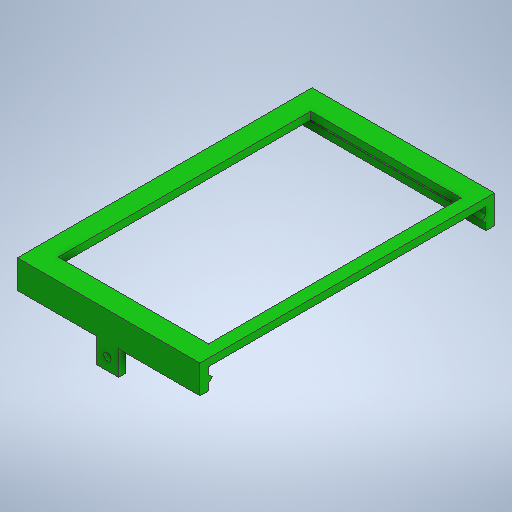
# Autodesk Inventor part: plate top
Saved by Autodesk Inventor 2026.1 (Build 301233020, 233B)
## iProperties
Created: 2025-07-03
Part Number: plate top
Material: Generic
Document SubType Name: Modeling
Designer: admin
Density: 1 g/cm^3
Appearance: Default
Author: admin
Autodesk Inventor part; units mm, degrees
ref_plane "YZ Plane" through (0, 0, 0) normal (1, 0, 0) x (0, 1, 0)
ref_plane "XZ Plane" through (0, 0, 0) normal (0, 1, 0) x (-1, 0, 0)
ref_plane "XY Plane" through (0, 0, 0) normal (0, 0, 1) x (1, 0, 0)
sketch "Sketch1" plane through (0, 0, 0) normal (0, 1, 0) x (-1, 0, 0)
  line L0 (21.9355, 25.495) -> (-52.0645, 25.495)
  line L1 (-52.0645, 25.495) -> (-52.0645, -94.005)
  line L2 (-52.0645, -94.005) -> (21.9355, -94.005)
  line L3 (21.9355, -94.005) -> (21.9355, 25.495)
  point P0 (0, 0)
  dimension "d0" = 119.5
  dimension "d1" = 74
  constraints: 8 end point, 3 perpendicular, 1 horizontal
  measures "d0" distance of L2.end L0.start
  measures "d1" distance of L0.start L0.end
extrude "Extrusion1" add sketch "Sketch1" against normal blind 3
sketch "Sketch2" plane through (0, 0, 0) normal (0, 1, 0) x (1, 0, 0)
  line L0 (-13.9355, -16.995) -> (-13.9355, 85.505)
  line L1 (-13.9355, 85.505) -> (47.0645, 85.505)
  line L2 (-21.9355, 94.005) -> (52.0645, 94.005) projected
  line L3 (47.0645, 85.505) -> (47.0645, -16.995)
  line L4 (47.0645, -16.995) -> (-13.9355, -16.995)
  line L5 (-21.9355, -25.495) -> (52.0645, -25.495) projected
  line L6 (-21.9355, 94.005) -> (-21.9355, -25.495) projected
  line L7 (52.0645, -25.495) -> (52.0645, 94.005) projected
  point P0 (0, 0)
  dimension "d4" = 8.5
  dimension "d5" = 8.5
  dimension "d6" = 8
  dimension "d7" = 5
  constraints: 8 end point, 2 perpendicular, 1 parallel, 1 vertical
  measures "d4" distance between parallel lines of L4 L5
  measures "d5" distance between parallel lines of L1 L2
  measures "d6" distance between parallel lines of L0 L6
  measures "d7" distance between parallel lines of L7 L3
extrude "Extrusion2" cut sketch "Sketch2" against normal blind 3 contours L0 L1 L3 L4
sketch "Sketch7" plane through (0, -3, 0) normal (0, -1, 0) x (1, 0, 0)
  line L0 (52.0645, 25.495) -> (-21.9355, 25.495) projected
  line L1 (52.0645, 25.495) -> (52.0645, 21.995)
  line L2 (52.0645, -94.005) -> (52.0645, 25.495) projected
  line L3 (52.0645, 21.995) -> (-21.9355, 21.995)
  line L4 (-21.9355, 21.995) -> (-21.9355, 25.495)
  line L5 (-21.9355, 25.495) -> (52.0645, 25.495)
  line L6 (52.0645, -94.005) -> (52.0645, -90.505)
  line L7 (52.0645, -90.505) -> (-21.9355, -90.505)
  line L8 (-21.9355, -90.505) -> (-21.9355, -94.005)
  line L9 (-21.9355, -94.005) -> (52.0645, -94.005)
  point P0 (0, 0)
  point P1 (-21.9355, 25.495)
  dimension "d82" = 3.5
  dimension "d83" = 74
  dimension "d84" = 3.5
  dimension "d107" = 74
  constraints: 16 end point, 6 perpendicular, 2 point on line
  measures "d82" distance of L0.start L1.end
  measures "d83" distance of L1.end L3.end
  measures "d84" distance of L2.start L6.end
  measures "d107" distance of L6.end L7.end
extrude "Extrusion7" add sketch "Sketch7" along normal blind 8.5
sketch "Sketch8" plane through (52.0645, 0, 25.495) normal (1, 0, 0) x (0, 0, -1)
  line L0 (3.5, -3) -> (3.5, -11.5) projected
  line L1 (3.5, -5.75) -> (5, -7.25)
  line L2 (5, -7.25) -> (3.5, -8.75)
  line L3 (116, -3) -> (3.5, -3) projected
  line L4 (116, -3) -> (116, -11.5) projected
  line L5 (116, -5.75) -> (114.5, -7.25)
  line L6 (114.5, -7.25) -> (116, -8.75)
  point P0 (25.495, 0)
  dimension "d87" = 45
  dimension "d88" = 1.5
  dimension "d89" = 4.25
  dimension "d90" = 45
  dimension "d91" = 45
  dimension "d92" = 4.25
  dimension "d93" = 1.5
  constraints: 8 end point, 4 point on line, 1 perpendicular
  measures "d87" angle of L1 L0
  measures "d88" distance from line of L0 L1.end
  measures "d89" distance from line of L3 L1.end
  measures "d90" angle of L4 L5
  measures "d91" angle of L4 L6
  measures "d92" distance from line of L3 L5.end
  measures "d93" distance from line of L5.end L4
extrude "Extrusion8" add sketch "Sketch8" against normal blind 74
sketch "Sketch9" plane through (0, -11.5, 0) normal (0, -1, 0) x (1, 0, 0)
  line L0 (-21.9355, 25.495) -> (52.0645, 25.495) projected
  line L1 (10.0645, 25.495) -> (19.0645, 25.495)
  line L2 (19.0645, 25.495) -> (19.0645, 22.495)
  line L3 (10.0645, 22.495) -> (10.0645, 25.495)
  line L4 (52.0645, 21.995) -> (52.0645, 25.495) projected
  line L5 (-21.9355, 25.495) -> (-21.9355, 21.995) projected
  line L6 (10.0645, 22.495) -> (19.0645, 22.495)
  line L7 (52.0645, 21.995) -> (-21.9355, 21.995) projected
  point P0 (0, 0)
  dimension "d96" = 9
  dimension "d97" = 3
  dimension "d99" = 32
  constraints: 8 end point, 2 parallel, 1 horizontal, 1 perpendicular, 1 point on line
  measures "d96" distance of L2.end L3.start
  measures "d97" distance of L1.end L2.end
  measures "d99" distance between parallel lines of L3 L5
extrude "Extrusion9" add sketch "Sketch9" along normal blind 10 contours L0 L2 L6 L3
sketch "Sketch10" plane through (-21.9355, 0, 25.495) normal (0, 0, 1) x (1, 0, 0)
  circle A0 centre (36.5, -16.5) radius 1.5
  line L0 (41, -21.5) -> (32, -21.5) projected
  line L1 (32, -11.5) -> (32, -21.5) projected
  point P0 (21.9355, 0)
  dimension "d102" = 3
  dimension "d103" = 5
  dimension "d104" = 4.5
  constraints: 1 centre point
  measures "d102" diameter of A0
  measures "d103" distance from line of A0.centre L0
  measures "d104" distance from line of L1 A0.centre
extrude "Extrusion10" cut sketch "Sketch10" against normal blind 10
body "Solid1"
